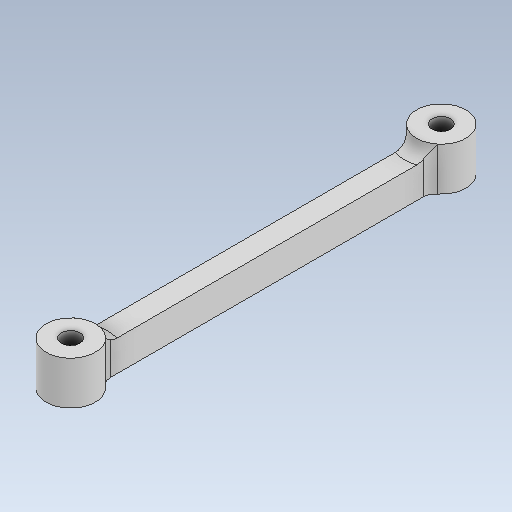
# Autodesk Inventor part: leg_link_3_m
Saved by Autodesk Inventor 2023 (Build 270158000, 158)
## iProperties
Created: 2020-12-12
Part Number: leg_link_3_m
Material: Generic
Document SubType Name: Modeling
Designer: Shuang Peng
Density: 1 g/cm^3
Appearance: Default
Author: Shuang Peng
Autodesk Inventor part; units mm, degrees
ref_plane "YZ Plane" through (0, 0, 0) normal (1, 0, 0) x (0, 1, 0)
ref_plane "XZ Plane" through (0, 0, 0) normal (0, 1, 0) x (-1, 0, 0)
ref_plane "XY Plane" through (0, 0, 0) normal (0, 0, 1) x (1, 0, 0)
sketch "Sketch1" plane through (0, 0, 0) normal (0, 1, 0) x (-1, 0, 0)
  circle A0 centre (0, 0) radius 4
  line L0 (0, 0) -> (0, -60)
  circle A1 centre (0, -60) radius 4
  line L1 (0, 0) -> (0, -60) construction
  line L2 (-1.75, 0) -> (-1.75, -60)
  line L3 (1.75, -60) -> (1.75, 0)
  arc A2 (1.75, 0) -> (-1.75, 0) centre (0, 0) ccw
  arc A3 (-1.75, -60) -> (1.75, -60) centre (0, -60) ccw
  point P0 (0, -30)
  point P1 (-1.75, -3.5969)
  point P2 (-1.75, -56.4031)
  point P3 (1.75, -56.4031)
  point P4 (1.75, -3.5969)
  dimension "d0" = 8
  dimension "d1" = 60
  dimension "d2" = 8
  dimension "d3" = 3.5
  constraints: 10 end point, 4 centre point, 4 point on circle, 4 tangent, 2 coincident, 2 equal length, 1 midpoint, 1 vertical
  measures "d0" diameter of A0
  measures "d1" distance of L0.start L0.end
  measures "d2" diameter of A1
  measures "d3" diameter of A3
extrude "Extrusion1" add sketch "Sketch1" along normal blind 7
sketch "Sketch2" plane through (0, 7, 0) normal (0, 1, 0) x (1, 0, 0)
  line L0 (1.75, 3.5969) -> (1.75, 56.4031) projected
  arc A0 (1.75, 56.4031) -> (-1.75, 56.4031) centre (0, 60) ccw projected
  line L1 (-1.75, 56.4031) -> (-1.75, 3.5969) projected
  arc A1 (-1.75, 3.5969) -> (1.75, 3.5969) centre (0, 0) ccw projected
  circle A2 centre (0, 0) radius 4
  circle A3 centre (0, 60) radius 4
  point P0 (-1.75, 56.4031)
  point P1 (-1.75, 3.5969)
  dimension "d6" = 8
  dimension "d7" = 8
  constraints: 2 centre point, 2 coincident
  measures "d6" diameter of A2
  measures "d7" diameter of A3
extrude "Extrusion2" cut sketch "Sketch2" against normal blind 2 contours A2 L1 A3 L0
sketch "Sketch3" plane through (0, 7, 0) normal (0, 1, 0) x (1, 0, 0)
  circle A0 centre (0, 0) radius 4 projected
  circle A1 centre (0, 60) radius 4 projected
hole "Hole1" at (0, 7, 0) at (0, 7, -60) direction (0, -1, 0) diameter 3 depth 8
fillet "Fillet1" radius 2 6 edges at (1.75, 2.5, -56.4031) (0, 5, -56) (-1.75, 2.5, -56.4031) (-1.75, 2.5, -3.5969) (0, 5, -4) (1.75, 2.5, -3.5969)
body "Solid1"
